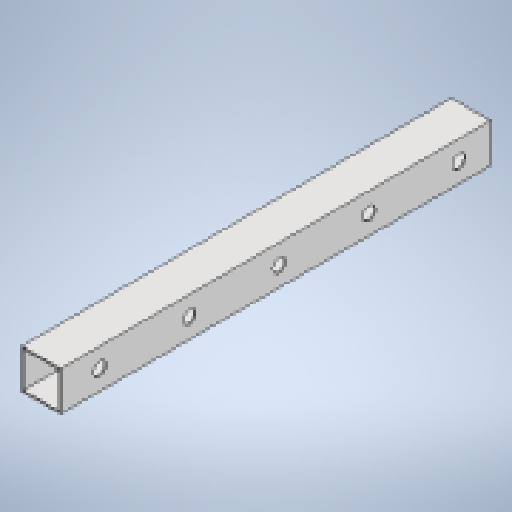
# Autodesk Inventor part: TKS 3511 FDS way tube 7
Saved by Autodesk Inventor 2025 (Build 290162010, 162A)
## iProperties
Created: 2025-06-24
Part Number: TKS 3511 FDS way tube 7
Material: Stainless Steel
Document SubType Name: Modeling
Designer: user
Mass: 1762.25 g
Surface Area: 2283.33 cm^2
Volume: 220.281 cm^3
Density: 8 g/cm^3
Sheet Metal Width: 0.000 mm
Sheet Metal Length: 0.000 mm
Sheet Metal Area: 0.000 mm^2
Appearance: Default
Sheet Metal Rule: AISI304 2mm Die16
Author: user
Autodesk Inventor part; units mm, degrees
ref_plane "YZ Plane" through (0, 0, 0) normal (1, 0, 0) x (0, 1, 0)
ref_plane "XZ Plane" through (0, 0, 0) normal (0, 1, 0) x (-1, 0, 0)
ref_plane "XY Plane" through (0, 0, 0) normal (0, 0, 1) x (1, 0, 0)
sketch "Sketch9" plane through (0, 0, 0) normal (0, 1, 0) x (-1, 0, 0)
  line L0 (25, 25) -> (-25, 25)
  line L1 (-25, 25) -> (-25, -25)
  line L2 (-25, -25) -> (25, -25)
  line L3 (25, -25) -> (25, 25)
  line L4 (25, 25) -> (-25, -25) construction
  line L5 (-25, 25) -> (25, -25) construction
  line L6 (-23, 23) -> (23, 23)
  line L7 (23, 23) -> (23, -23)
  line L8 (23, -23) -> (-23, -23)
  line L9 (-23, -23) -> (-23, 23)
  point P0 (0, 0)
  dimension "d172" = 50
  dimension "d173" = 50
  dimension "d174" = 2
  constraints: 20 end point, 4 parallel, 2 midpoint, 2 perpendicular, 1 horizontal, 3 other
  measures "d172" distance of L2.end L1.end
  measures "d173" distance of L0.end L1.end
  measures "d174" distance between parallel lines of L0 L6
extrude "Extrusion3" add sketch "Sketch9" against normal blind 515
sketch "Sketch10" plane through (0, 0, 0) normal (1, 0, 0) x (0, 1, 0)
  line L0 (0, 25) -> (0, -25) construction
  line L1 (0, 25) -> (-515, 25) construction
  line L2 (-515, -25) -> (-515, 25) construction
  line L3 (0, -25) -> (-515, -25) construction
  line L4 (-48.5, 8.5) -> (-31.5, 8.5)
  line L5 (-31.5, 8.5) -> (-31.5, -8.5)
  line L6 (-31.5, -8.5) -> (-48.5, -8.5)
  line L7 (-48.5, -8.5) -> (-48.5, 8.5)
  line L8 (-48.5, 8.5) -> (-31.5, -8.5) construction
  line L9 (-31.5, 8.5) -> (-48.5, -8.5) construction
  line L10 (-163.5, 8.5) -> (-146.5, 8.5)
  line L11 (-146.5, 8.5) -> (-146.5, -8.5)
  line L12 (-146.5, -8.5) -> (-163.5, -8.5)
  line L13 (-163.5, -8.5) -> (-163.5, 8.5)
  line L14 (-163.5, 8.5) -> (-146.5, -8.5) construction
  line L15 (-146.5, 8.5) -> (-163.5, -8.5) construction
  line L16 (-278.5, 8.5) -> (-261.5, 8.5)
  line L17 (-261.5, 8.5) -> (-261.5, -8.5)
  line L18 (-261.5, -8.5) -> (-278.5, -8.5)
  line L19 (-278.5, -8.5) -> (-278.5, 8.5)
  line L20 (-278.5, 8.5) -> (-261.5, -8.5) construction
  line L21 (-261.5, 8.5) -> (-278.5, -8.5) construction
  circle A0 centre (-500, 0) radius 8.5
  line L22 (0, 0) -> (40, 0)
  circle A1 centre (-40, 0) radius 8.5
  circle A2 centre (-155, 0) radius 8.5
  circle A3 centre (-270, 0) radius 8.5
  line L23 (-376.5, -8.5) -> (-393.5, -8.5)
  line L24 (-393.5, -8.5) -> (-393.5, 8.5)
  line L25 (-393.5, 8.5) -> (-376.5, 8.5)
  line L26 (-376.5, 8.5) -> (-376.5, -8.5)
  line L27 (-376.5, -8.5) -> (-393.5, 8.5) construction
  line L28 (-393.5, -8.5) -> (-376.5, 8.5) construction
  circle A4 centre (-385, 0) radius 8.5
  dimension "d177" = 17
  dimension "d178" = 17
  dimension "d181" = 40
  dimension "d182" = 80
  dimension "d185" = 540
  dimension "d186" = 17
  dimension "d188" = 460
  dimension "d189" = 115
  dimension "d190" = 115
  dimension "d191" = 115
  constraints: 50 end point, 9 midpoint, 8 parallel, 5 centre point, 5 horizontal, 5 horizontal alignment, 5 tangent, 4 coincident, 4 perpendicular, 3 equal length, 1 equal radius, 1 point on line
  measures "d177" distance of L4.start L4.end
  measures "d178" distance of L4.end L5.end
  measures "d181" distance of L22.start L22.end
  measures "d182" distance of point (-40, 0) L22.end
  measures "d185" distance of L22.end A0.centre
  measures "d186" diameter of A0
  measures "d188" distance of A0.centre point (-40, 0)
  measures "d189" distance of point (-155, 0) point (-40, 0)
  measures "d190" distance of point (-270, 0) point (-155, 0)
  measures "d191" distance of A3.centre point (-385, 0)
extrude "Extrusion4" cut sketch "Sketch10" along normal through all contours A1 | A2 | A3 | A0 | A4
body "Solid4"
